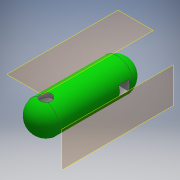
# Autodesk Inventor part: brazopalo
Saved by Autodesk Inventor 2016 (Build 200138000, 138)
## iProperties
Created: 2016-02-20
Part Number: brazopalo
Material: Genérico
Document SubType Name: Modeling
Designer: Usuario1
Density: 1 g/cm^3
Appearance: Valor por defecto
Author: Usuario1
Autodesk Inventor part; units mm, degrees
ref_plane "XZ Plane" through (0, 0, 0) normal (0, 1, 0) x (-1, 0, 0)
sketch "Boceto1" plane through (0, 0, 0) normal (0, 0, 1) x (1, 0, 0)
  line L0 (-1.2847, 1.0744) -> (-1.2847, 7.0094)
  line L1 (-0.9847, 1.1029) -> (-0.9847, 6.9809)
  arc A0 (-1.2847, 1.0744) -> (0, 0) centre (0, 1.3052) ccw
  arc A1 (-0.9847, 1.1029) -> (0, 0.3) centre (0, 1.3052) ccw
  arc A2 (0, 8.0838) -> (-1.2847, 7.0094) centre (0, 6.7786) ccw
  arc A3 (0, 7.7838) -> (-0.9847, 6.9809) centre (0, 6.7786) ccw
  line L2 (0, 0.3) -> (0, 0)
  line L3 (0, 7.7838) -> (0, 8.0838)
  line L4 (0, 7.7838) -> (0, 5.2838)
  line L5 (0, 5.2838) -> (-0.9847, 5.2838)
  line L6 (-0.9847, 6.9809) -> (-0.9847, 5.2838)
  point P0 (0, 0)
  dimension "d2" = 2.5
  constraints: 14 end point, 8 point on circle, 4 centre point, 1 collinear, 1 perpendicular, 1 point on line, 1 vertical
  measures "d2" distance of L3.start L4.end
revolve "Revolución1" add sketch "Boceto1" angle 360 about axis through (0, 0.3, 0) along (0, -1, 0)
ref_plane "Plano de trabajo1" through (3, 0, 0) normal (1, 0, 0) x (0, 1, 0)
sketch "Boceto2" plane through (3, 0, 0) normal (1, 0, 0) x (0, 1, 0)
  line L0 (1.0744, 1.2847) -> (7.0094, 1.2847)
  line L1 (1.1029, 0.9847) -> (6.9809, 0.9847)
  arc A0 (1.0744, 1.2847) -> (0, 0) centre (1.3052, 0) ccw
  arc A1 (1.1029, 0.9847) -> (0.3, 0) centre (1.3052, 0) ccw
  arc A2 (8.0838, 0) -> (7.0094, 1.2847) centre (6.7786, 0) ccw
  arc A3 (7.7838, 0) -> (6.9809, 0.9847) centre (6.7786, 0) ccw
  line L2 (6.7094, 0.4) -> (6.7094, -0.4)
  line L3 (5.9094, -0.4) -> (5.9094, 0.4)
  line L4 (0.3, 0) -> (0, 0)
  line L5 (7.7838, 0) -> (8.0838, 0)
  line L6 (6.7094, 0.4) -> (5.9094, 0.4)
  line L7 (6.7094, -0.4) -> (5.9094, -0.4)
  constraints: 16 end point, 8 point on circle, 4 centre point
extrude "Extrusión1" cut sketch "Boceto2" against normal blind 3 contours L2 L7 L3 L6
ref_plane "Plano de trabajo2" through (0, 0, 3) normal (0, 0, 1) x (1, 0, 0)
sketch "Boceto3" plane through (0, 0, 3) normal (0, 0, 1) x (1, 0, 0)
  line L0 (-1.2847, 1.0744) -> (-1.2847, 7.0094)
  line L1 (-0.9847, 1.1029) -> (-0.9847, 6.9809)
  arc A0 (-1.2847, 1.0744) -> (0, 0) centre (0, 1.3052) ccw
  arc A1 (-0.9847, 1.1029) -> (0, 0.3) centre (0, 1.3052) ccw
  arc A2 (0, 8.0838) -> (-1.2847, 7.0094) centre (0, 6.7786) ccw
  arc A3 (0, 7.7838) -> (-0.9847, 6.9809) centre (0, 6.7786) ccw
  line L2 (0, 0.3) -> (0, 0)
  line L3 (0, 7.7838) -> (0, 8.0838)
  circle A4 centre (0, 1.3052) radius 0.45
  point P0 (0, 0)
  constraints: 8 end point, 8 point on circle, 5 centre point
extrude "Extrusión2" cut sketch "Boceto3" against normal blind 8 contours A4
